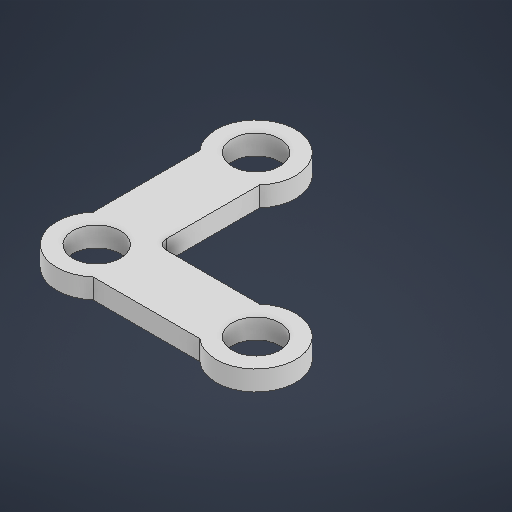
# Autodesk Inventor part: link-1-turn-8
Saved by Autodesk Inventor 2025.4 (Build 294407000, 407)
## iProperties
Created: 2026-09-15
Part Number: link-1-turn-8
Material: Generic
Document SubType Name: Modeling
Designer: User
Density: 1 g/cm^3
Appearance: Default
Author: User
Autodesk Inventor part; units mm, degrees
ref_plane "YZ Plane" through (0, 0, 0) normal (1, 0, 0) x (0, 1, 0)
ref_plane "XZ Plane" through (0, 0, 0) normal (0, 1, 0) x (-1, 0, 0)
ref_plane "XY Plane" through (0, 0, 0) normal (0, 0, 1) x (1, 0, 0)
sketch "Sketch1" plane through (0, 0, 0) normal (0, 1, 0) x (-1, 0, 0)
  line L0 (-1.5, -4) -> (1.5, -4)
  line L1 (1.5, -4) -> (1.5, 4)
  line L2 (1.5, 4) -> (-1.5, 4)
  line L3 (-1.5, 2) -> (-1.5, -4)
  line L4 (-1.5, -4) -> (1.5, 4) construction
  line L5 (1.5, -4) -> (-1.5, 4) construction
  circle A0 centre (0, 4) radius 1.2
  circle A1 centre (0, -4) radius 1.2
  circle A2 centre (0, -4) radius 2
  circle A3 centre (0, 4) radius 2
  line L6 (-2, 2.5) -> (-8, 2.5)
  line L7 (-8, 2.5) -> (-8, 5.5)
  line L8 (-8, 5.5) -> (0, 5.5)
  line L9 (0, 5.5) -> (0, 2.5)
  circle A4 centre (-8, 4) radius 1.2
  circle A5 centre (-8, 4) radius 2
  arc A6 (-1.5, 2) -> (-2, 2.5) centre (-2, 2) ccw
  point P0 (0, 0)
  point P1 (-1.5, -2.6771)
  point P2 (1.5, -2.6771)
  point P3 (1.5, 2.6771)
  point P4 (-1.5, 2.6771)
  point P5 (-6.6771, 2.5)
  point P6 (-1.5, 2.5)
  point P7 (-1.3229, 5.5)
  point P8 (-6.6771, 5.5)
  point P9 (-8, 5.2)
  point P10 (-8, 2.8)
  dimension "d0" = 3
  dimension "linkPitchLength" = 8
  dimension "d3" = 2.4
  dimension "d4" = 4
  dimension "linkPitchWidth" = 8
  dimension "d17" = 0.5
  constraints: 20 end point, 7 centre point, 6 midpoint, 4 equal radius, 4 parallel, 3 coincident, 3 perpendicular, 2 horizontal, 2 point on circle, 2 point on line, 2 tangent
  measures "d0" distance of L2.end L1.end
  measures "linkPitchLength" distance of L1.end L0.end
  measures "d3" diameter of A1
  measures "d4" diameter of A2
  measures "linkPitchWidth" distance between parallel lines of L7 L9
  measures "d17" radius of A6
extrude "Extrusion1" add sketch "Sketch1" along normal blind 1 contours A1 L0 L3 A2 L1 | L0 L1 A2 L3 A1 | A2 L3 A6 L6 A5 L8 A3 L1 | A3 L8 L9 A0 L2 L1 | L1 L2 A0 L9 L8 A3 | A5 L6 L7 A4 L8 | L8 L7 A4 L6 A5
sketch "Sketch2" plane through (0, 1, 0) normal (0, 1, 0) x (1, 0, 0)
  line L0 (6.6771, -2.5) -> (2, -2.5) projected
  arc A0 (1.5, -2) -> (2, -2.5) centre (2, -2) ccw projected
  line L1 (1.5, -2) -> (1.5, 2.6771) projected
  arc A1 (1.5, 2.6771) -> (-1.5, 2.6771) centre (0, 4) ccw projected
  line L2 (-1.5, 2.6771) -> (-1.5, -2.6771) projected
  arc A2 (-1.5, -2.6771) -> (1.3229, -5.5) centre (0, -4) ccw projected
  line L3 (1.3229, -5.5) -> (6.6771, -5.5) projected
  arc A3 (6.6771, -5.5) -> (6.6771, -2.5) centre (8, -4) ccw projected
  circle A4 centre (8, -4) radius 1.2 projected
  circle A5 centre (0, 4) radius 1.2 projected
  circle A6 centre (0, -4) radius 1.2 projected
  point P0 (0, 0)
extrude "Extrusion2" [suppressed]
sketch "Sketch5" plane through (0, 1, 0) normal (0, 1, 0) x (1, 0, 0)
  line L0 (6.6771, -2.5) -> (2, -2.5) projected
  arc A0 (1.5, -2) -> (2, -2.5) centre (2, -2) ccw projected
  line L1 (1.5, -2) -> (1.5, 2.6771) projected
  arc A1 (1.5, 2.6771) -> (-1.5, 2.6771) centre (0, 4) ccw projected
  line L2 (-1.5, 2.6771) -> (-1.5, -2.6771) projected
  arc A2 (-1.5, -2.6771) -> (1.3229, -5.5) centre (0, -4) ccw projected
  line L3 (1.3229, -5.5) -> (6.6771, -5.5) projected
  arc A3 (6.6771, -5.5) -> (6.6771, -2.5) centre (8, -4) ccw projected
  circle A4 centre (8, -4) radius 1.2 projected
  circle A5 centre (0, 4) radius 1.2 projected
  circle A6 centre (0, -4) radius 1.2 projected
  point P0 (0, 0)
extrude "Extrusion3" [suppressed]
sketch "Sketch6" plane through (0, 1, 0) normal (0, 1, 0) x (1, 0, 0)
  line L0 (6.6771, -2.5) -> (2, -2.5) projected
  arc A0 (1.5, -2) -> (2, -2.5) centre (2, -2) ccw projected
  line L1 (1.5, -2) -> (1.5, 2.6771) projected
  arc A1 (1.5, 2.6771) -> (-1.5, 2.6771) centre (0, 4) ccw projected
  line L2 (-1.5, 2.6771) -> (-1.5, -2.6771) projected
  arc A2 (-1.5, -2.6771) -> (1.3229, -5.5) centre (0, -4) ccw projected
  line L3 (1.3229, -5.5) -> (6.6771, -5.5) projected
  arc A3 (6.6771, -5.5) -> (6.6771, -2.5) centre (8, -4) ccw projected
  circle A4 centre (8, -4) radius 1.2 projected
  circle A5 centre (0, 4) radius 1.2 projected
  circle A6 centre (0, -4) radius 1.2 projected
  point P0 (0, 0)
extrude "Extrusion4" [suppressed]
body "Solid1"
